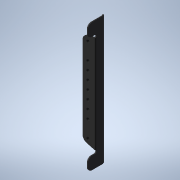
# Autodesk Inventor part: 1301.000_3_(1)
Saved by Autodesk Inventor 2021 (Build 250183000, 183)
## iProperties
Created: 2025-05-02
Part Number: 1301.000_3_(1)
Material: Generic
Catalog Web Link: www.cadenas.de
Description: Seitenteil KX EB Edelstahl-Seitenteil KX EB Edelstahl
Vendor: RITTAL
Document SubType Name: Modeling
Designer: psAdmin
Manufacturer: RITTAL
Mass: 8.11983 g
Surface Area: 118.905 cm^2
Volume: 8.11983 cm^3
Density: 1 g/cm^3
Appearance: PSOLRGB-175-175-175
Category: PARTsolutions
Company: RITTAL
Title: 1301.000_3
Author: Cadenas PARTsolutions
Comments: Seitenteil KX EB Edelstahl
PSOL_IDENT_0: {$CADENAS_DATA/23d-libs/rittal/schaltschranksys/edelstahl/kleingehause/parts_eb_edel_2_0/seitenteil_
PSOL_IDENT_1: kx_eb_edel_new.prj},197 {VTYP=3D},{NB=1301.000_3_(1)},{LINA=1301.000_3},{NN=Seitenteil KX EB Edelsta
PSOL_IDENT_2: hl},{DATE=28.04.2025 21:10:48},{GEOMDATE=11.04.2025 11:21:29},{VERSION=},{LINEID=370},{WBVAR=DETAIL}
PSOL_IDENT_3: ,{WBNUMERIC=DETAIL}  {NB=1301.000_3_(1)},{LINA=1301.000_3},{KT=DUMMY},{BEST=1301.000},{DETAIL=1},{H1=
PSOL_IDENT_4: 50},{BEZ1=Klemmenkästen KL},{BEZ2=ohne Flansch},{BEZ3=Stahlblech},{VER=2},{VERS=2},{X=4},{CNSETIM40=
PSOL_IDENT_5: EC002713},{CNSECLASS51=27-18-01-02},{CNSECLASS70=27-18-01-01},{CNSECLASS80=27-18-01-01},{GEW=3,889},
PSOL_IDENT_6: {CNSETIM80=EC000261},{CNSETIM90=EC000261},{CNSECLASS60=27-18-01-01},{UNSPSC=31-26-15-02}
NB: 1301.000_3_(1)
NN: Seitenteil KX EB Edelstahl
NT: Seitenteil KX EB Edelstahl
NBSYN: $BEST._3_($DETAIL.)
LINA: 1301.000_3
CATALOG: Rittal
BEST: 1301.000
DETAIL: hoch
H1: 50
BEZ1: Klemmenkästen KL
BEZ2: ohne Flansch
BEZ3: Stahlblech
VER: 2
VERS: 2
X: 4
CNSECLASS70: 27-18-01-01
CNSECLASS80: 27-18-01-01
GEW: 3,889
CNSETIM80: EC000261
CNSETIM90: EC000261
CNSECLASS60: 27-18-01-01
UNSPSC: 31-26-15-02
SUPPLIER: RITTAL
ARTICLENO: 1301.000_3_(1)
BOMINFO: 1301.000_3
CREATOR: CADENAS GmbH
Autodesk Inventor part; units mm, degrees
sketch "Sketch_1" plane through (0, 0, 0) normal (0, 1, 0) x (-1, 0, 0)
  line L0 (19, -2) -> (19, 0)
  line L1 (19, 0) -> (1.5, 0)
  line L2 (1.5, 0) -> (1.5, 11)
  line L3 (1.5, 11) -> (0, 11)
  line L4 (0, 11) -> (0, -10.471)
  arc A0 (0, -10.471) -> (0.1809, -11.4971) centre (3, -10.471) ccw
  line L5 (0.1809, -11.4971) -> (1.0919, -14)
  line L6 (1.0919, -14) -> (2.5014, -13.487)
  line L7 (2.5014, -13.487) -> (1.5905, -10.984)
  arc A1 (1.5, -10.471) -> (1.5905, -10.984) centre (3, -10.471) ccw
  line L8 (1.5, -10.471) -> (1.5, -2)
  line L9 (1.5, -2) -> (19, -2)
  constraints: 20 end point, 4 point on circle, 2 centre point
extrude "Extrusion1" add sketch "Sketch_1" along normal mid plane 190
sketch "Sketch_2" plane through (0, 0, 0) normal (1, 0, 0) x (0, 1, 0)
  line L0 (-71, 79.5) -> (-71, 73)
  line L1 (-71, 73) -> (-76.5, 67.5)
  line L2 (-76.5, 67.5) -> (-76.5, 1)
  arc A0 (-76.5, 1) -> (-71.7087, 0) centre (-74, 1) ccw
  line L3 (-71.7087, 0) -> (71.7087, 0)
  arc A1 (71.7087, 0) -> (76.5, 1) centre (74, 1) ccw
  line L4 (76.5, 1) -> (76.5, 67.5)
  line L5 (76.5, 67.5) -> (71, 73)
  line L6 (71, 73) -> (71, 79.5)
  line L7 (71, 79.5) -> (-71, 79.5)
  constraints: 16 end point, 4 point on circle, 2 centre point
extrude "Extrusion2" cut sketch "Sketch_2" along normal mid plane 110
sketch "Sketch_3" plane through (0, 0, 0) normal (1, 0, 0) x (0, 1, 0)
  line L0 (-105, 90) -> (-105, -20)
  line L1 (-105, -20) -> (105, -20)
  line L2 (105, -20) -> (105, 90)
  line L3 (105, 90) -> (-105, 90)
  arc A0 (-89, 11) -> (-95, 5) centre (-89, 5) ccw
  line L4 (-95, 5) -> (-95, -15)
  line L5 (-95, -15) -> (95, -15)
  line L6 (95, -15) -> (95, 5)
  arc A1 (95, 5) -> (89, 11) centre (89, 5) ccw
  line L7 (89, 11) -> (82.5, 11)
  arc A2 (82.5, 11) -> (76.5, 5) centre (82.5, 5) ccw
  line L8 (76.5, 5) -> (76.5, 4)
  line L9 (76.5, 4) -> (-76.5, 4)
  line L10 (-76.5, 4) -> (-76.5, 5)
  arc A3 (-76.5, 5) -> (-82.5, 11) centre (-82.5, 5) ccw
  line L11 (-82.5, 11) -> (-89, 11)
  constraints: 24 end point, 8 point on circle, 4 centre point
extrude "Extrusion3" cut sketch "Sketch_3" along normal mid plane 110
sketch "Sketch_5" plane through (0, 0, 0) normal (0, 0, 1) x (1, 0, 0)
  line L0 (-21.5, 125) -> (-21.5, -125)
  line L1 (-21.5, -125) -> (-1.5, -125)
  line L2 (-1.5, -125) -> (-1.5, -74)
  arc A0 (-1.5, -74) -> (-3.353, -71.5852) centre (-4, -74) ccw
  line L3 (-3.353, -71.5852) -> (-13.0706, -68.9814)
  arc A1 (-19, -61.254) -> (-13.0706, -68.9814) centre (-11, -61.254) ccw
  line L4 (-19, -61.254) -> (-19, 61.254)
  arc A2 (-13.0706, 68.9814) -> (-19, 61.254) centre (-11, 61.254) ccw
  line L5 (-13.0706, 68.9814) -> (-3.353, 71.5852)
  arc A3 (-3.353, 71.5852) -> (-1.5, 74) centre (-4, 74) ccw
  line L6 (-1.5, 74) -> (-1.5, 125)
  line L7 (-1.5, 125) -> (-21.5, 125)
  constraints: 16 end point, 8 point on circle, 4 centre point
extrude "Extrusion4" cut sketch "Sketch_5" along normal mid plane 5
sketch "Sketch_91" plane through (0, 0, 0) normal (0, 0, 1) x (1, 0, 0)
  line L0 (-19, 67.3926) -> (-19, -67.3926)
  line L1 (-19, -67.3926) -> (-1.5, -72.0817)
  line L2 (-1.5, -72.0817) -> (0, -72.0817)
  line L3 (0, -72.0817) -> (0, 72.0817)
  line L4 (0, 72.0817) -> (-1.5, 72.0817)
  line L5 (-1.5, 72.0817) -> (-19, 67.3926)
  constraints: 12 end point
extrude "Extrusion5" add sketch "Sketch_91" against normal blind 2.5
sketch "Sketch_6" plane through (0, 0, 0) normal (0, 1, 0) x (-1, 0, 0)
  line L0 (1.5, 0) -> (1.5, 3.5)
  line L1 (1.5, 3.5) -> (-3.5, 3.5)
  line L2 (-3.5, 3.5) -> (-3.5, -1.5)
  line L3 (-3.5, -1.5) -> (0, -1.5)
  arc A0 (1.5, 0) -> (0, -1.5) centre (1.5, -1.5) ccw
  constraints: 8 end point, 2 point on circle, 1 centre point
extrude "Extrusion6" cut sketch "Sketch_6" along normal mid plane 148
sketch "Sketch_9" plane through (0, 0, 0) normal (0, 1, 0) x (-1, 0, 0)
  line L0 (21.5, -6.5) -> (21.5, -1.5)
  line L1 (21.5, -1.5) -> (1.5, -1.5)
  line L2 (1.5, -1.5) -> (1.5, -6.5)
  line L3 (1.5, -6.5) -> (21.5, -6.5)
  constraints: 8 end point
extrude "Extrusion7" cut sketch "Sketch_9" along normal mid plane 196
sketch "Sketch_7" plane through (-11, 0, 0) normal (1, 0, 0) x (0, 0, -1)
  line L0 (0, 62.5) -> (3.2, 62.5)
  line L1 (3.2, 62.5) -> (3.2, 59.25)
  line L2 (3.2, 59.25) -> (1.8, 59.25)
  arc A0 (1.8, 59.25) -> (1.5, 58.95) centre (1.8, 58.95) ccw
  line L3 (1.5, 58.95) -> (0, 59.25)
  line L4 (0, 59.25) -> (0, 62.5)
  line L5 (0, 62.5) -> (3.2, 62.5)
  constraints: 12 end point, 2 point on circle, 1 centre point
revolve "Revolution1" add sketch "Sketch_7" angle 360 about axis through (-11, 62.5, 0) along (0, 0, 1)
pattern_linear "Rectangular Pattern1" count 11 spacing 12.5 along (0, -1, 0) of "Revolution1"
sketch "Sketch9" plane through (-19, -67.3926, 0) normal (0, 0, 1) x (1, 0, 0)
  point P0 (8, 129.8926)
hole "Hole1" at (-11, 62.5, 0) direction (0, 0, -1) diameter 4.6 depth 3.2
pattern_linear "Rectangular Pattern2" count 11 spacing 12.5 along (0, -1, 0) of "Hole1"
sketch "Sketch_105" plane through (0, 0, 0) normal (0, 0, 1) x (1, 0, 0)
  line L0 (-17, -45) -> (-17, -55)
  line L1 (-17, -55) -> (-3, -55)
  line L2 (-3, -55) -> (-3, 55)
  line L3 (-3, 55) -> (-17, 55)
  line L4 (-17, 55) -> (-17, 45)
  line L5 (-17, 45) -> (-6, 45)
  line L6 (-6, 45) -> (-6, -45)
  line L7 (-6, -45) -> (-17, -45)
  constraints: 16 end point
extrude "Extrusion8" add sketch "Sketch_105" against normal blind 1.5
sketch "Sketch_106" plane through (0, 0, -1.5) normal (0, 0, 1) x (1, 0, 0)
  line L0 (-17, -45) -> (-17, -55)
  line L1 (-17, -55) -> (-3, -55)
  line L2 (-3, -55) -> (-3, 55)
  line L3 (-3, 55) -> (-17, 55)
  line L4 (-17, 55) -> (-17, 45)
  line L5 (-17, 45) -> (-6, 45)
  line L6 (-6, 45) -> (-6, -45)
  line L7 (-6, -45) -> (-17, -45)
  constraints: 16 end point
extrude "Extrusion9" cut sketch "Sketch_106" against normal blind 1.7
fillet "Fillet1" radius 8 2 edges at (-19, 67.3926, -0.75) (-19, -67.3926, -0.75)
ref_plane "SC1_XY" through (-11, 25, 0) normal (0, 0, -1) x (1, 0, 0)
ref_plane "SC1_YZ" through (-11, 25, 0) normal (1, 0, 0) x (0, -1, 0)
ref_plane "SC1_ZX" through (-11, 25, 0) normal (0, -1, 0) x (0, 0, -1)
ref_plane "SC2_XY" through (-11, -25, 0) normal (0, 0, -1) x (1, 0, 0)
ref_plane "SC2_YZ" through (-11, -25, 0) normal (1, 0, 0) x (0, -1, 0)
ref_plane "SC2_ZX" through (-11, -25, 0) normal (0, -1, 0) x (0, 0, -1)
ref_plane "SEITENTEIL_XY" through (0, 0, 0) normal (-1, 0, 0) x (0, 0, -1)
ref_plane "SEITENTEIL_YZ" through (0, 0, 0) normal (0, 0, -1) x (0, -1, 0)
ref_plane "SEITENTEIL_ZX" through (0, 0, 0) normal (0, -1, 0) x (-1, 0, 0)
body "Solid1"
